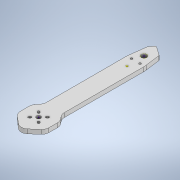
# Autodesk Inventor part: og kauri arm
Saved by Autodesk Inventor 2020 (Build 240168000, 168)
## iProperties
Created: 2022-08-12
Part Number: og kauri arm
Material: Generic
Document SubType Name: Modeling
Designer: Steven
Density: 1 g/cm^3
Appearance: Default
Author: Steven
Autodesk Inventor part; units mm, degrees
ref_plane "YZ Plane" through (0, 0, 0) normal (1, 0, 0) x (0, 1, 0)
ref_plane "XZ Plane" through (0, 0, 0) normal (0, 1, 0) x (-1, 0, 0)
ref_plane "XY Plane" through (0, 0, 0) normal (0, 0, 1) x (1, 0, 0)
sketch "Sketch1" plane through (0, 0, 0) normal (0, 1, 0) x (-1, 0, 0)
  circle A0 centre (0.4121, -148.477) radius 4
  arc A1 (9.1115, -162.2046) -> (9.3712, -161.5303) centre (7.8828, -161.3443) ccw
  line L0 (9.1115, -162.2046) -> (4.9561, -168.1392)
  arc A2 (2.867, -168.5075) -> (4.9561, -168.1392) centre (3.7274, -167.2788) ccw
  line L1 (2.867, -168.5075) -> (-9.0439, -160.1674)
  arc A3 (-9.6719, -159.1247) -> (-9.0439, -160.1674) centre (-8.1835, -158.9387) ccw
  line L2 (-9.6719, -159.1247) -> (-12.2297, -138.6622)
  arc A4 (-12.5, -134.321) -> (-12.2297, -138.6622) centre (22.5, -134.321) ccw
  line L3 (-12.5, -134.321) -> (-12.5, -23.3333)
  arc A5 (-12.5, -23.3333) -> (-14.5, -17.3333) centre (-22.5, -23.3333) ccw
  line L4 (-14.5, -17.3333) -> (-18, -12.6667)
  arc A6 (-20, -6.6667) -> (-18, -12.6667) centre (-10, -6.6667) ccw
  line L5 (-20, -6.6667) -> (-20, 5.4953)
  arc A7 (-16.6262, 12.9849) -> (-20, 5.4953) centre (-10, 5.4953) ccw
  line L6 (-16.6262, 12.9849) -> (-6.6262, 21.8321)
  arc A8 (6.6262, 21.8321) -> (-6.6262, 21.8321) centre (0, 14.3426) ccw
  line L7 (6.6262, 21.8321) -> (16.6262, 12.9849)
  arc A9 (20, 5.4953) -> (16.6262, 12.9849) centre (10, 5.4953) ccw
  line L8 (20, 5.4953) -> (20, -6.6667)
  arc A10 (18, -12.6667) -> (20, -6.6667) centre (10, -6.6667) ccw
  line L9 (18, -12.6667) -> (14.5, -17.3333)
  arc A11 (14.5, -17.3333) -> (12.5, -23.3333) centre (22.5, -23.3333) ccw
  line L10 (12.5, -23.3333) -> (12.5, -134.321)
  arc A12 (12.2297, -138.6622) -> (12.5, -134.321) centre (-22.5, -134.321) ccw
  line L11 (12.2297, -138.6622) -> (9.3712, -161.5303)
  arc A13 (-7.7782, -5.6569) -> (-5.6569, -7.7782) centre (-6.7175, -6.7175) ccw
  line L12 (-7.7782, -5.6569) -> (-6.7175, -4.5962)
  arc A14 (-4.5962, -6.7175) -> (-6.7175, -4.5962) centre (-5.6569, -5.6569) ccw
  line L13 (-4.5962, -6.7175) -> (-5.6569, -7.7782)
  circle A15 centre (-6, -136.5) radius 1.5
  circle A16 centre (6, -136.5) radius 1.5
  arc A17 (5.6569, -7.7782) -> (7.7782, -5.6569) centre (6.7175, -6.7175) ccw
  line L14 (5.6569, -7.7782) -> (4.5962, -6.7175)
  arc A18 (6.7175, -4.5962) -> (4.5962, -6.7175) centre (5.6569, -5.6569) ccw
  line L15 (6.7175, -4.5962) -> (7.7782, -5.6569)
  circle A19 centre (0, -124.0736) radius 1.5
  line L16 (6.7175, 4.5962) -> (7.7782, 5.6569)
  arc A20 (7.7782, 5.6569) -> (5.6569, 7.7782) centre (6.7175, 6.7175) ccw
  line L17 (5.6569, 7.7782) -> (4.5962, 6.7175)
  arc A21 (4.5962, 6.7175) -> (6.7175, 4.5962) centre (5.6569, 5.6569) ccw
  circle A22 centre (0, 0) radius 3
  arc A23 (-6.7175, 4.5962) -> (-4.5962, 6.7175) centre (-5.6569, 5.6569) ccw
  line L18 (-6.7175, 4.5962) -> (-7.7782, 5.6569)
  arc A24 (-5.6569, 7.7782) -> (-7.7782, 5.6569) centre (-6.7175, 6.7175) ccw
  line L19 (-5.6569, 7.7782) -> (-4.5962, 6.7175)
  point P0 (12.5, -23.3333)
  point P1 (14.5, -17.3333)
  point P2 (16.6262, 12.9849)
  point P3 (6.6262, 21.8321)
  point P4 (-6.6262, 21.8321)
  point P5 (-18, -12.6667)
  point P6 (-12.5, -23.3333)
  point P7 (4.9561, -168.1392)
  point P8 (7.7782, -5.6569)
  point P9 (5.6569, -7.7782)
  point P10 (4.5962, -6.7175)
  point P11 (6.7175, 4.5962)
  point P12 (-7.7782, 5.6569)
  point P13 (-5.6569, 7.7782)
  point P14 (-4.5962, -6.7175)
  point P15 (-5.6569, -7.7782)
  constraints: 40 end point, 40 point on circle, 25 centre point
extrude "Extrusion1" add sketch "Sketch1" along normal blind 6
sketch "Sketch2" plane through (0, 6, 0) normal (0, 1, 0) x (1, 0, 0)
  circle A0 centre (0, 124.0736) radius 1.5 construction
  circle A1 centre (-0.4121, 148.477) radius 4 construction
  point P0 (0, 0)
body "Solid1"
